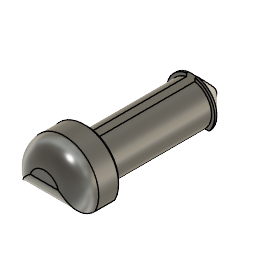
2mm pin (Autodesk Fusion 360 design; units mm, degrees)
Autodesk Fusion 360 part; units mm, degrees
note: some values were not read from the file. Chosen so that the rebuilt part matches the saved one: which face or edge a step refers to; which pieces of a blend or face edit are solid. Set by a fixed rule: which sketch regions a step uses.
sketch "Sketch1" plane through (0, 0, 0) normal (0, 1, 0) x (1, 0, 0)
  circle A0 centre (0, 0) radius 1
  line L0 (0, 0) -> (0, 1)
  line L1 (0, 0.5) -> (0, 1)
  line L2 (0, 0.75) -> (0.6614, 0.75)
  line L3 (0, 0.75) -> (-0.6614, 0.75)
  line L4 (0, 1) -> (-0.2, 1)
  line L5 (-0.2, 1) -> (0.2, 1)
  line L6 (0.2, 1) -> (0.2, -1)
  line L7 (0.2, -1) -> (-0.2, -1)
  line L8 (-0.2, -1) -> (-0.2, 1)
  circle A1 centre (0, 0) radius 1.15
  line L9 (-0.6614, 0.75) -> (-0.8718, 0.75)
  line L10 (0.6614, 0.75) -> (0.8718, 0.75)
  line L11 (0.2, -1) -> (0.2, -1.1325)
  line L12 (-0.2, -1) -> (-0.2, -1.1325)
  dimension "d1" = 2
  dimension "d2" = 0.2
  dimension "d3" = 0.4
  dimension "d4" = 2
  dimension "d5" = 2.3
  constraint coincident A0.centre L0.start
  constraint coincident A0 L0.end
  constraint vertical L0
  constraint midpoint L0 L1.start
  constraint midpoint L1 L2.start
  constraint coincident A0 L2.end
  constraint perpendicular L1 L2
  constraint coincident A0 L3.end
  constraint perpendicular L1 L3
  constraint perpendicular L1 L4
  constraint horizontal L5
  constraint vertical L6
  constraint horizontal L7
  constraint vertical L8
  constraint coincident A1 L9.end
  constraint parallel L3 L9
  constraint coincident A1 L10.end
  constraint parallel L2 L10
  constraint coincident A1 L11.end
  constraint perpendicular L7 L11
  constraint coincident A1 L12.end
  constraint perpendicular L7 L12
  measures "d1" diameter of A0
  measures "d2" distance of L0.end L4.end
  measures "d3" distance of L4.end L5.end
  measures "d4" distance of L4.end L7.end
  measures "d5" diameter of A1
extrude "Extrude1" add sketch "Sketch1" against normal blind 2 contours A0 L2 L6 | A0 L6 A1 L10 L11 | A0 L6 L7 | A0 L2 L3 L6 L8 | A0 L7 L8 | L7 A1 L11 L12 | A0 L8 A1 L9 L12 | A0 L3 L8 picked at (0.244, -0.391) picked at (-0.2474, -0.3898)
extrude "Extrude2" add sketch "Sketch1" along normal blind 5 contours A0 L2 L6 | A0 L3 L8 picked at (0.244, -0.391) picked at (-0.2474, -0.3898)
extrude "Extrude3" add sketch "Sketch1" along normal blind 1 from surface at 5 contours A0 L2 L6 | A0 L6 A1 L10 L11 | A0 L8 A1 L9 L12 | A0 L3 L8 picked at (0.244, -0.391) picked at (-0.2474, -0.3898)
move_face "OffsetFaces1" offset 0.5 1 faces at (-1.0727, -0.6667, 0.4146)
chamfer "Chamfer1" distance 0.9 angle 45 4 edges at (-1.0831, 6, 0.3865) (1.0831, 6, 0.3865) (0.5359, 6, -0.75) (-0.5359, 6, -0.75)
fillet "Fillet1" radius 0.95 1 faces at (-0.2331, -2, -0.0019)
chamfer "Chamfer2" distance 0.1 angle 45 1 edges at (0, 0, 1.65)
